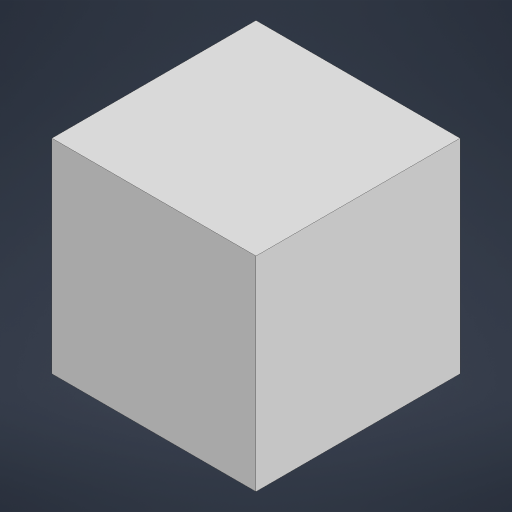
# Autodesk Inventor part: Powietrze
Saved by Autodesk Inventor 2023 (Build 270158000, 158)
## iProperties
Created: 2023-02-10
Part Number: Powietrze
Material: Generic
Document SubType Name: Modeling
Designer: szykr
Density: 1 g/cm^3
Appearance: Default
Author: szykr
Autodesk Inventor part; units mm, degrees
ref_plane "YZ Plane" through (0, 0, 0) normal (1, 0, 0) x (0, 1, 0)
ref_plane "XZ Plane" through (0, 0, 0) normal (0, 1, 0) x (-1, 0, 0)
ref_plane "XY Plane" through (0, 0, 0) normal (0, 0, 1) x (1, 0, 0)
sketch "Sketch1" plane through (0, 0, 0) normal (0, 1, 0) x (-1, 0, 0)
  line L0 (-2000, 2000) -> (2000, 2000)
  line L1 (2000, 2000) -> (2000, -2000)
  line L2 (2000, -2000) -> (-2000, -2000)
  line L3 (-2000, -2000) -> (-2000, 2000)
  line L4 (-2000, 2000) -> (2000, -2000) construction
  line L5 (2000, 2000) -> (-2000, -2000) construction
  point P0 (0, 0)
  dimension "d0" = 4000
  dimension "d1" = 4000
  constraints: 12 end point, 2 midpoint, 2 parallel, 1 horizontal, 1 perpendicular
  measures "d0" distance of L1.end L2.end
  measures "d1" distance of L0.end L1.end
extrude "Extrusion1" add sketch "Sketch1" along normal mid plane 4000
body "Solid1"
